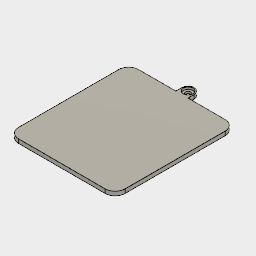
CaseV2 Back Cover v3 (Autodesk Fusion 360 design; units mm, degrees)
Autodesk Fusion 360 part; units mm, degrees
note: some values were not read from the file. Set by a fixed rule: which face or edge a step refers to.
sketch "Sketch1" plane through (0, 0, 0) normal (0, 1, 0) x (1, 0, 0)
  line L0 (26.4985, -29.7) -> (-26.4985, -29.7)
  line L1 (-26.4985, -29.7) -> (-26.4985, 29.7)
  line L2 (-26.4985, 29.7) -> (26.4985, 29.7)
  line L3 (26.4985, 29.7) -> (26.4985, -29.7)
  line L4 (26.4985, -29.7) -> (-26.4985, 29.7) construction
  line L5 (-26.4985, -29.7) -> (26.4985, 29.7) construction
  line L6 (3, 29.7) -> (-3, 29.7)
  line L7 (-3, 29.7) -> (-3, 32.7)
  line L8 (-3, 32.7) -> (3, 32.7)
  line L9 (3, 32.7) -> (3, 29.7)
  line L10 (3, 29.7) -> (-3, 32.7) construction
  line L11 (-3, 29.7) -> (3, 32.7) construction
  arc A0 (3, 32.7) -> (-3, 32.7) centre (0, 32.7) ccw
  circle A1 centre (0, 32.7) radius 1.25
  point P0 (0, 31.2)
  dimension "d1" = 52.997
  dimension "d2" = 59.4
  dimension "d3" = 6
  dimension "d4" = 3
  dimension "d5" = 2.5
  measures "d1" distance of L1.end L2.end
  measures "d2" distance of L0.end L1.end
  measures "d3" distance of L7.end L8.end
  measures "d4" distance of L6.end L7.end
  measures "d5" diameter of A1
extrude "Extrude1" add sketch "Sketch1" along normal blind 2 contours L0 L1 L2 L3 L6 | L2 L6 L7 L8 L9 A1 | L8 A0 A1
sketch "Sketch2" plane through (0, 2, 0) normal (0, 1, 0) x (-1, 0, 0)
  circle A0 centre (0, -32.7) radius 1.25
  line L0 (-3, -29.7) -> (-3, -32.7)
  arc A1 (-3, -32.7) -> (3, -32.7) centre (0, -32.7) ccw
  line L1 (3, -32.7) -> (3, -29.7)
  line L2 (3, -29.7) -> (26.4985, -29.7)
  line L3 (26.4985, -29.7) -> (26.4985, 29.7)
  line L4 (26.4985, 29.7) -> (-26.4985, 29.7)
  line L5 (-26.4985, 29.7) -> (-26.4985, -29.7)
  line L6 (-26.4985, -29.7) -> (-3, -29.7)
  circle A2 centre (0, -32.7) radius 2.4
  dimension "d8" = 4.8
  measures "d8" diameter of A2
extrude "Extrude2" cut sketch "Sketch2" against normal blind 1.4 contours A2
extrude "Extrude3" add 1 faces at (-2.0031, 0.6, -32.8813) along direction (0, 1, 0) blind 0.4
fillet "Fillet1" chord length 7 4 edges at (-26.4985, 1, -29.7) (26.4985, 1, -29.7) (26.4985, 1, 29.7) (-26.4985, 1, 29.7)
move_face "OffsetFaces1" offset -0.25 1 faces at (-26.4985, 0.6667, 8.2501)
move_face "OffsetFaces2" offset -0.25 1 faces at (26.4985, 1.3333, 8.2501)
move_face "OffsetFaces3" offset -0.25 1 faces at (7.0996, 0.6667, 29.7)
